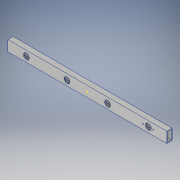
# Autodesk Inventor part: 30inchbarchassis
Saved by Autodesk Inventor 2019 (Build 230136000, 136)
## iProperties
Created: 2019-01-12
Part Number: 30inchbarchassis
Material: Aluminum 6061
Document SubType Name: Modeling
Designer: lebraddock
Density: 2.7 g/cm^3
Appearance: Aluminum - Flat
Mass: 856.952 g
Surface Area: 2038.6 cm^2
Volume: 317.39 cm^3
Author: lebraddock
Autodesk Inventor part; units mm, degrees
ref_plane "YZ Plane" through (0, 0, 0) normal (1, 0, 0) x (0, 1, 0)
ref_plane "XZ Plane" through (0, 0, 0) normal (0, 1, 0) x (-1, 0, 0)
ref_plane "XY Plane" through (0, 0, 0) normal (0, 0, 1) x (1, 0, 0)
sketch "Sketch1" plane through (0, 0, 0) normal (0, 0, 1) x (1, 0, 0)
  line L0 (-381, -25.4) -> (381, -25.4)
  line L1 (381, -25.4) -> (381, 25.4)
  line L2 (381, 25.4) -> (-381, 25.4)
  line L3 (-381, 25.4) -> (-381, -25.4)
  line L4 (-381, -25.4) -> (381, 25.4) construction
  line L5 (381, -25.4) -> (-381, 25.4) construction
  point P0 (0, 0)
  dimension "d0" = 762
  dimension "d1" = 50.8
  constraints: 12 end point, 2 midpoint, 2 parallel, 1 horizontal, 1 perpendicular
  measures "d0" distance of L2.end L1.end
  measures "d1" distance of L1.end L0.end
extrude "Extrusion1" add sketch "Sketch1" along normal blind 25.4
sketch "Sketch2" plane through (381, -25.4, 0) normal (1, 0, 0) x (0, 0, -1)
  line L0 (-25.4, 0) -> (-25.4, 50.8) projected
  line L1 (-25.4, 50.8) -> (0, 50.8)
  line L2 (0, 50.8) -> (0, 0)
  line L3 (0, 0) -> (-25.4, 0)
  line L4 (-25.4, 0) -> (-25.4, 50.8)
  line L5 (-3.175, 47.625) -> (-22.225, 47.625)
  line L6 (-22.225, 47.625) -> (-22.225, 3.175)
  line L7 (-22.225, 3.175) -> (-3.175, 3.175)
  line L8 (-3.175, 3.175) -> (-3.175, 47.625)
  point P0 (0, 25.4)
  dimension "d4" = 3.175
  constraints: 16 end point, 4 parallel, 2 perpendicular, 1 horizontal, 3 other
  measures "d4" distance between parallel lines of L1 L5
extrude "Extrusion2" cut sketch "Sketch2" against normal blind 762 contours L8 L7 L6 L5
sketch "Sketch3" plane through (0, 0, 25.4) normal (0, 0, 1) x (1, 0, 0)
  circle A0 centre (-292.5356, 0) radius 14.2875
  circle A1 centre (292.5356, 0) radius 14.2875
  line L0 (381, 25.4) -> (-381, 25.4) projected
  line L1 (0, 25.4) -> (0, -25.4)
  line L2 (-381, -25.4) -> (381, -25.4) projected
  dimension "d40" = 292.5356
  dimension "d41" = 292.5356
  constraints: 2 centre point, 2 end point, 2 midpoint
  measures "d40" distance from line of L1 A0.centre
  measures "d41" distance from line of L1 A1.centre
extrude "Extrusion3" cut sketch "Sketch3" against normal blind 25.4
sketch "Sketch5" plane through (0, 0, 25.4) normal (0, 0, 1) x (1, 0, 0)
  point P0 (0, 0)
sketch "Sketch6" plane through (0, 0, 25.4) normal (0, 0, 1) x (1, 0, 0)
  circle A0 centre (97.4989, -1.5875) radius 14.2875
  circle A1 centre (-97.4989, -1.5875) radius 14.2875
  line L0 (381, 25.4) -> (-381, 25.4) projected
  point P0 (0, 0)
  dimension "d28" = 97.5119
  dimension "d29" = 97.5119
  dimension "d30" = 28.575
  dimension "d31" = 28.575
  dimension "d34" = 26.9875
  dimension "d35" = 26.9875
  constraints: 2 centre point
  measures "d28" distance of point (0, 0) A0.centre
  measures "d29" distance of point (0, 0) A1.centre
  measures "d30" diameter of A0
  measures "d31" diameter of A1
  measures "d34" distance from line of L0 A0.centre
  measures "d35" distance from line of L0 A1.centre
extrude "Extrusion5" cut sketch "Sketch6" against normal blind 25.4
sketch "Sketch8" plane through (0, 0, 25.4) normal (0, 0, 1) x (1, 0, 0)
  circle A0 centre (268.7231, 0) radius 2.413
  circle A1 centre (316.3481, 0) radius 2.413
  circle A2 centre (292.5356, 0) radius 14.2875 projected
  point P0 (0, 0)
  dimension "d42" = 47.625
  dimension "d43" = 23.8125
  dimension "d44" = 4.826
  dimension "d45" = 4.826
  constraints: 2 centre point
  measures "d42" distance of A0.centre A1.centre
  measures "d43" distance of A2.centre A0.centre
  measures "d44" diameter of A1
  measures "d45" diameter of A0
extrude "Extrusion7" cut sketch "Sketch8" against normal blind 25.4 contours A0 | A1
body "Solid1"
